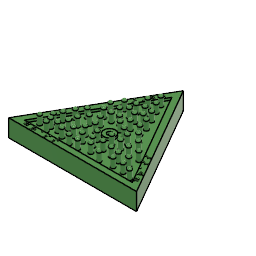
Piece Grass (Autodesk Fusion 360 design; units mm, degrees)
Autodesk Fusion 360 part; units mm, degrees
sketch "Sketch1" plane through (0, 0, 0) normal (0, 1, 0) x (1, 0, 0) in component "Peice Base"
  line L0 (0, 0) -> (69.85, 120.9837)
  line L1 (0, 0) -> (139.7, 0)
  line L2 (69.85, 120.9837) -> (139.7, 0)
  dimension "d1" = 139.7
  dimension "d2" = 139.7
  dimension "d4" = 139.7
  constraint coincident L0.start L1.start
  constraint horizontal L1
  measures "d1" distance of L0.start L0.end
  measures "d2" distance of L0.start L1.end
  measures "d4" distance of L0.end L1.end
extrude "Extrude1" add sketch "Sketch1" along normal blind 19.05 makes body 1 in component "Peice Base"
sketch "Sketch1 (2)" plane through (0, 0, 0) normal (0, 1, 0) x (1, 0, 0) in component "grass"
  line L0 (0, 0) -> (69.85, 120.9837)
  line L1 (0, 0) -> (139.7, 0)
  line L2 (69.85, 120.9837) -> (139.7, 0)
  dimension "d1_1" = 139.7
  dimension "d2_1" = 139.7
  dimension "d4_1" = 139.7
  constraint coincident L0.start L1.start
  constraint horizontal L1
  measures "d1_1" distance of L0.start L0.end
  measures "d2_1" distance of L0.start L1.end
  measures "d4_1" distance of L0.end L1.end
extrude "Extrude1'" add sketch "Sketch1 (2)" along normal blind 19.05 separate body makes body 2 in component "grass"
sketch "Sketch5" plane through (0, 19.05, 0) normal (0, 1, 0) x (-1, 0, 0) in component "grass"
  line L0 (0, 0) -> (-139.7, 0)
  line L1 (-139.7, 0) -> (-69.85, -120.9837)
  line L2 (-69.85, -120.9837) -> (0, 0)
  line L3 (-128.7015, -6.35) -> (-69.85, -108.2837)
  line L4 (-69.85, -108.2837) -> (-10.9985, -6.35)
  line L5 (-10.9985, -6.35) -> (-128.7015, -6.35)
  circle A0 centre (-69.85, -40.3279) radius 2.54
  circle A1 centre (-69.85, -40.3279) radius 6.35
  circle A2 centre (-69.537, -96.6095) radius 2.286
  circle A3 centre (-64.3272, -87.6271) radius 2.286
  circle A4 centre (-73.4892, -87.6271) radius 2.286
  circle A5 centre (-63.2493, -76.1296) radius 2.286
  circle A6 centre (-58.0395, -63.1949) radius 2.286
  circle A7 centre (-70.9742, -66.6083) radius 2.286
  circle A8 centre (-78.8787, -77.2075) radius 2.286
  circle A9 centre (-70.6149, -78.2854) radius 2.286
  circle A10 centre (-83.7292, -66.6083) radius 2.286
  circle A11 centre (-85.7053, -57.6258) radius 2.286
  circle A12 centre (-75.4654, -57.3169) radius 2.286
  circle A13 centre (-65.2254, -56.009) radius 2.286
  circle A14 centre (-49.596, -54.2125) radius 2.286
  circle A15 centre (-53.5483, -72.896) radius 2.286
  circle A16 centre (-40.4243, -45.4098) radius 2.286
  circle A17 centre (-55.7041, -44.5115) radius 2.286
  circle A18 centre (-79.4176, -46.6673) radius 2.286
  circle A19 centre (-92.1727, -49.7213) radius 2.286
  circle A20 centre (-58.9377, -35.7087) radius 2.286
  circle A21 centre (-48.1588, -40.0203) radius 2.286
  circle A22 centre (-34.925, -37.8645) radius 2.286
  circle A23 centre (-99.5383, -42.1761) radius 2.286
  circle A24 centre (-87.3222, -42.3557) radius 2.286
  circle A25 centre (-79.0583, -33.553) radius 2.286
  circle A26 centre (-88.7594, -33.553) radius 2.286
  circle A27 centre (-87.8611, -10.9173) radius 2.286
  circle A28 centre (-101.1551, -12.8934) radius 2.286
  circle A29 centre (-90.3762, -21.6962) radius 2.286
  circle A30 centre (-99.179, -31.7565) radius 2.286
  circle A31 centre (-99.3586, -20.4386) radius 2.286
  circle A32 centre (-112.1136, -12.8934) radius 2.286
  circle A33 centre (-109.4189, -21.8758) radius 2.286
  circle A34 centre (-109.4189, -32.8344) radius 2.286
  circle A35 centre (-121.4554, -10.558) radius 2.286
  circle A36 centre (-30.5533, -28.7025) radius 2.286
  circle A37 centre (-43.488, -31.9361) radius 2.286
  circle A38 centre (-56.4227, -27.2653) radius 2.286
  circle A39 centre (-67.7405, -29.0618) radius 2.286
  circle A40 centre (-80.1362, -22.9537) radius 2.286
  circle A41 centre (-75.4654, -14.3306) radius 2.286
  circle A42 centre (-70.7945, -21.1572) radius 2.286
  circle A43 centre (-61.0935, -19.3607) radius 2.286
  circle A44 centre (-64.6865, -10.558) radius 2.286
  circle A45 centre (-55.5244, -10.558) radius 2.286
  circle A46 centre (-51.0332, -19.8997) radius 2.286
  circle A47 centre (-41.5118, -23.852) radius 2.286
  circle A48 centre (-29.9275, -16.0295) radius 2.286
  circle A49 centre (-27.14, -21.6962) radius 2.286
  circle A50 centre (-37.7392, -15.9474) radius 2.286
  circle A51 centre (-45.2845, -12.8934) radius 2.286
  circle A52 centre (-71.1538, -50.6196) radius 2.286
  circle A53 centre (-47.9792, -63.1949) radius 2.286
  circle A54 centre (-76.7229, -70.2012) radius 2.286
  circle A55 centre (-57.6802, -54.3922) radius 2.286
  circle A56 centre (-63.2493, -68.5844) radius 2.286
  circle A57 centre (-20.5941, -13.3685) radius 2.286
  circle A58 centre (-30.8095, -10.3039) radius 2.286
  circle A59 centre (-14.8274, -5.4566) radius 0.7493
  circle A60 centre (-17.1134, -5.4566) radius 0.7493
  circle A61 centre (-17.1134, -3.1706) radius 0.7493
  circle A62 centre (-14.8274, -3.1706) radius 0.7493
  circle A63 centre (-23.2348, -5.4566) radius 0.7493
  circle A64 centre (-23.2348, -3.1706) radius 0.7493
  circle A65 centre (-23.2348, -0.8846) radius 0.7493
  circle A66 centre (-25.5208, -3.1706) radius 0.7493
  circle A67 centre (-31.6422, -5.4566) radius 0.7493
  circle A68 centre (-37.7636, -3.1706) radius 0.7493
  circle A69 centre (-37.7636, -0.8846) radius 0.7493
  circle A70 centre (-40.0496, -5.4566) radius 0.7493
  circle A71 centre (-40.0496, -5.4566) radius 0.7493
  circle A72 centre (-46.171, -3.1706) radius 0.7493
  circle A73 centre (-46.171, -0.8846) radius 0.7493
  circle A74 centre (-48.457, -5.4566) radius 0.7493
  circle A75 centre (-118.2703, -30.7774) radius 0.7493
  circle A76 centre (-115.1476, -31.6141) radius 0.7493
  circle A77 centre (-128.5954, -12.8938) radius 0.7493
  circle A78 centre (-116.0464, -39.2014) radius 0.7493
  circle A79 centre (-110.9439, -38.8951) radius 0.7493
  circle A80 centre (-125.5347, -18.195) radius 0.7493
  circle A81 centre (-119.3513, -24.3331) radius 0.7493
  circle A82 centre (-115.1476, -31.6141) radius 0.7493
  circle A83 centre (-129.7384, -10.914) radius 0.7493
  circle A84 centre (-120.2501, -31.9204) radius 0.7493
  circle A85 centre (-123.555, -17.052) radius 0.7493
  circle A86 centre (-126.6157, -11.7508) radius 0.7493
  circle A87 centre (-114.0666, -38.0584) radius 0.7493
  circle A88 centre (-124.3917, -20.1748) radius 0.7493
  circle A89 centre (-127.7587, -9.771) radius 0.7493
  circle A90 centre (-127.5145, -19.338) radius 0.7493
  circle A91 centre (-52.8628, -85.2716) radius 0.7493
  circle A92 centre (-53.6996, -82.1488) radius 0.7493
  circle A93 centre (-63.1879, -103.1551) radius 0.7493
  circle A94 centre (-46.6794, -79.1335) radius 0.7493
  circle A95 centre (-49.4959, -74.8678) radius 0.7493
  circle A96 centre (-60.1272, -97.8539) radius 0.7493
  circle A97 centre (-57.9033, -89.4298) radius 0.7493
  circle A98 centre (-53.6996, -82.1488) radius 0.7493
  circle A99 centre (-64.3309, -105.1349) radius 0.7493
  circle A100 centre (-50.8831, -86.4146) radius 0.7493
  circle A101 centre (-62.107, -96.7109) radius 0.7493
  circle A102 centre (-65.1677, -102.0121) radius 0.7493
  circle A103 centre (-48.6591, -77.9905) radius 0.7493
  circle A104 centre (-58.9842, -95.8741) radius 0.7493
  circle A105 centre (-66.3107, -103.9919) radius 0.7493
  circle A106 centre (-58.1475, -98.9969) radius 0.7493
  dimension "d22" = -6.35
  dimension "d40" = 5.08
  dimension "d41" = 69.85
  dimension "d42" = 40.3279
  dimension "d65" = 12.7
  dimension "d89" = 4.572
  dimension "d90" = 4.572
  dimension "d91" = 4.572
  dimension "d92" = 4.572
  dimension "d93" = 4.572
  dimension "d94" = 4.572
  dimension "d95" = 4.572
  dimension "d96" = 4.572
  dimension "d97" = 4.572
  dimension "d98" = 4.572
  dimension "d99" = 4.572
  dimension "d100" = 4.572
  dimension "d101" = 4.572
  dimension "d102" = 4.572
  dimension "d103" = 4.572
  dimension "d104" = 4.572
  dimension "d105" = 4.572
  dimension "d106" = 4.572
  dimension "d107" = 4.572
  dimension "d108" = 4.572
  dimension "d109" = 4.572
  dimension "d110" = 4.572
  dimension "d111" = 4.572
  dimension "d112" = 4.572
  dimension "d113" = 4.572
  dimension "d114" = 4.572
  dimension "d115" = 4.572
  dimension "d116" = 4.572
  dimension "d117" = 4.572
  dimension "d118" = 4.572
  dimension "d119" = 4.572
  dimension "d120" = 4.572
  dimension "d121" = 4.572
  dimension "d122" = 4.572
  dimension "d123" = 4.572
  dimension "d124" = 4.572
  dimension "d125" = 4.572
  dimension "d126" = 4.572
  dimension "d127" = 4.572
  dimension "d128" = 4.572
  dimension "d129" = 4.572
  dimension "d130" = 4.572
  dimension "d131" = 4.572
  dimension "d132" = 4.572
  dimension "d133" = 4.572
  dimension "d134" = 4.572
  dimension "d136" = 4.572
  dimension "d137" = 4.572
  dimension "d138" = 4.572
  dimension "d139" = 4.572
  dimension "d140" = 4.572
  dimension "d141" = 4.572
  dimension "d142" = 4.572
  dimension "d143" = 4.572
  dimension "d144" = 4.572
  dimension "d148" = 4.572
  dimension "d149" = 4.572
  dimension "d150" = 1.4986
  dimension "d151" = 1.4986
  dimension "d152" = 1.4986
  dimension "d153" = 1.4986
  dimension "d154" = 1.4986
  dimension "d155" = 1.4986
  dimension "d156" = 1.4986
  dimension "d157" = 1.4986
  dimension "d159" = 1.4986
  dimension "d160" = 1.4986
  dimension "d161" = 1.4986
  dimension "d163" = 1.4986
  dimension "d164" = 1.4986
  dimension "d166" = 1.4986
  dimension "d167" = 1.4986
  dimension "d169" = 1.4986
  dimension "d170" = 1.4986
  dimension "d171" = 1.4986
  dimension "d172" = 1.4986
  dimension "d173" = 1.4986
  dimension "d174" = 1.4986
  dimension "d175" = 1.4986
  dimension "d176" = 1.4986
  dimension "d177" = 1.4986
  dimension "d178" = 1.4986
  dimension "d179" = 1.4986
  dimension "d180" = 1.4986
  dimension "d181" = 1.4986
  dimension "d182" = 1.4986
  dimension "d183" = 1.4986
  dimension "d184" = 1.4986
  dimension "d185" = 1.4986
  dimension "d186" = 1.4986
  dimension "d187" = 1.4986
  dimension "d188" = 1.4986
  dimension "d189" = 1.4986
  dimension "d190" = 1.4986
  dimension "d191" = 1.4986
  dimension "d192" = 1.4986
  dimension "d193" = 1.4986
  dimension "d194" = 1.4986
  dimension "d195" = 1.4986
  dimension "d196" = 1.4986
  dimension "d197" = 1.4986
  dimension "d198" = 1.4986
  dimension "d199" = 1.4986
  dimension "d200" = 1.4986
  dimension "d201" = 1.4986
  constraint concentric A0 A1
  measures "d40" diameter of A0
  measures "d41" horizontal distance of L0.start A0.centre
  measures "d42" distance of L0 A0.centre
  measures "d65" diameter of A1
  measures "d89" diameter of A2
  measures "d90" diameter of A3
  measures "d91" diameter of A4
  measures "d92" diameter of A5
  measures "d93" diameter of A6
  measures "d94" diameter of A7
  measures "d95" diameter of A8
  measures "d96" diameter of A9
  measures "d97" diameter of A10
  measures "d98" diameter of A11
  measures "d99" diameter of A12
  measures "d100" diameter of A13
  measures "d101" diameter of A14
  measures "d102" diameter of A15
  measures "d103" diameter of A16
  measures "d104" diameter of A17
  measures "d105" diameter of A18
  measures "d106" diameter of A19
  measures "d107" diameter of A20
  measures "d108" diameter of A21
  measures "d109" diameter of A22
  measures "d110" diameter of A23
  measures "d111" diameter of A24
  measures "d112" diameter of A25
  measures "d113" diameter of A26
  measures "d114" diameter of A27
  measures "d115" diameter of A28
  measures "d116" diameter of A29
  measures "d117" diameter of A30
  measures "d118" diameter of A31
  measures "d119" diameter of A32
  measures "d120" diameter of A33
  measures "d121" diameter of A34
  measures "d122" diameter of A35
  measures "d123" diameter of A36
  measures "d124" diameter of A37
  measures "d125" diameter of A38
  measures "d126" diameter of A39
  measures "d127" diameter of A40
  measures "d128" diameter of A41
  measures "d129" diameter of A42
  measures "d130" diameter of A43
  measures "d131" diameter of A44
  measures "d132" diameter of A45
  measures "d133" diameter of A46
  measures "d134" diameter of A47
  measures "d136" diameter of A48
  measures "d137" diameter of A49
  measures "d138" diameter of A50
  measures "d139" diameter of A51
  measures "d140" diameter of A52
  measures "d141" diameter of A53
  measures "d142" diameter of A54
  measures "d143" diameter of A55
  measures "d144" diameter of A56
  measures "d148" diameter of A57
  measures "d149" diameter of A58
  measures "d150" diameter of A59
  measures "d151" diameter of A60
  measures "d152" diameter of A61
  measures "d153" diameter of A62
  measures "d154" diameter of A63
  measures "d155" diameter of A64
  measures "d156" diameter of A65
  measures "d157" diameter of A66
  measures "d159" diameter of A67
  measures "d160" diameter of A68
  measures "d161" diameter of A69
  measures "d163" diameter of A70
  measures "d164" diameter of A71
  measures "d166" diameter of A72
  measures "d167" diameter of A73
  measures "d169" diameter of A74
  measures "d170" diameter of A89
  measures "d171" diameter of A86
  measures "d172" diameter of A77
  measures "d173" diameter of A83
  measures "d174" diameter of A85
  measures "d175" diameter of A80
  measures "d176" diameter of A90
  measures "d177" diameter of A88
  measures "d178" diameter of A81
  measures "d179" diameter of A75
  measures "d180" diameter of A84
  measures "d181" diameter of A76
  measures "d182" diameter of A82
  measures "d183" diameter of A87
  measures "d184" diameter of A78
  measures "d185" diameter of A79
  measures "d186" diameter of A105
  measures "d187" diameter of A102
  measures "d188" diameter of A93
  measures "d189" diameter of A99
  measures "d190" diameter of A101
  measures "d191" diameter of A96
  measures "d192" diameter of A106
  measures "d193" diameter of A104
  measures "d194" diameter of A97
  measures "d195" diameter of A91
  measures "d196" diameter of A100
  measures "d197" diameter of A92
  measures "d198" diameter of A98
  measures "d199" diameter of A103
  measures "d200" diameter of A94
  measures "d201" diameter of A95
extrude "Extrude7" cut sketch "Sketch5" against normal blind 3.048 contours A0 bodies 2 in component "grass"
extrude "Extrude8" cut sketch "Sketch5" against normal blind 2.54 contours L3 L4 L5 bodies 2 in component "grass"
extrude "Extrude9" add sketch "Sketch5" along normal blind 8.89 contours A2 | A3 | A4 | A5 | A6 | A7 | A8 | A9 | A10 | A11 | A12 | A13 | A14 | A15 | A16 | A17 | A18 | A19 | A20 | A21 | A22 | A23 | A24 | A25 | A26 | A27 | A28 | A29 | A30 | A31 | A32 | A33 | A34 | A35 | A36 | A37 | A38 | A39 | A40 | A41 | A42 | A43 | A44 | A45 | A46 | A47 | A48 | A49 | A50 | A51 | A52 | A53 | A54 | A55 | A56 | A57 | A58 bodies 2 in component "grass"
fillet "Fillet1" radius 2.286 57 edges at (123.5867, 27.94, -11.3846) (114.2449, 27.94, -13.7201) (103.2864, 27.94, -13.7201) (89.9924, 27.94, -11.7439) (77.5967, 27.94, -15.1572) (66.8178, 27.94, -11.3846) (57.6557, 27.94, -11.3846) (63.2248, 27.94, -20.1874) (72.9258, 27.94, -21.9839) (82.2675, 27.94, -23.7804) (92.5075, 27.94, -22.5228) (101.4899, 27.94, -21.2653) (111.5502, 27.94, -22.7025) (111.5502, 27.94, -33.661) (101.3103, 27.94, -32.5831) (90.8907, 27.94, -34.3796) (89.4535, 27.94, -43.1824) (94.304, 27.94, -50.548) (101.6696, 27.94, -43.0027) (87.8366, 27.94, -58.4525) (85.8605, 27.94, -67.4349) (77.5967, 27.94, -58.1435) (81.1896, 27.94, -34.3796) (69.8718, 27.94, -29.8884) (58.554, 27.94, -28.0919) (53.1645, 27.94, -20.7263) (47.4158, 27.94, -13.7201) (32.9408, 27.94, -11.1306) (32.0588, 27.94, -16.8562) (22.7254, 27.94, -14.1952) (29.2713, 27.94, -22.5228) (32.6846, 27.94, -29.5291) (43.6431, 27.94, -24.6786) (39.8705, 27.94, -16.7741) (45.6193, 27.94, -32.7628) (37.0563, 27.94, -38.6912) (42.5556, 27.94, -46.2364) (50.2901, 27.94, -40.847) (57.8354, 27.94, -45.3382) (61.069, 27.94, -36.5354) (51.7273, 27.94, -55.0392) (50.1105, 27.94, -64.0216) (60.1708, 27.94, -64.0216) (59.8115, 27.94, -55.2188) (55.6796, 27.94, -73.7226) (67.3567, 27.94, -56.8357) (73.2851, 27.94, -51.4462) (81.5489, 27.94, -47.4939) (73.1055, 27.94, -67.4349) (65.3806, 27.94, -69.411) (65.3806, 27.94, -76.9563) (66.4585, 27.94, -88.4538) (75.6205, 27.94, -88.4538) (72.7462, 27.94, -79.1121) (81.01, 27.94, -78.0342) (78.8542, 27.94, -71.0279) (71.6683, 27.94, -97.4362) on bodies 2 in component "grass"
extrude "Extrude10" add sketch "Sketch5" along normal blind 0.762 contours A59 | A60 | A61 | A62 | A63 | A64 | A65 | A66 | A67 | A68 | A69 | A70 A71 | A72 | A73 | A74 | A75 | A76 A82 | A77 | A78 | A79 | A80 | A81 | A83 | A84 | A85 | A86 | A87 | A88 | A89 | A90 | A91 | A92 A98 | A93 | A94 | A95 | A96 | A97 | A99 | A100 | A101 | A102 | A103 | A104 | A105 | A106 bodies 2 in component "grass"
fillet "Fillet2" radius 0.7493 45 edges at (66.196, 19.812, -103.2514) (65.053, 19.812, -101.2717) (63.0733, 19.812, -102.4147) (64.2163, 19.812, -104.3944) (61.9923, 19.812, -95.9704) (58.8696, 19.812, -95.1336) (60.0126, 19.812, -97.1134) (58.0329, 19.812, -98.2564) (57.7886, 19.812, -88.6894) (50.7685, 19.812, -85.6741) (52.7482, 19.812, -84.5311) (53.5849, 19.812, -81.4083) (46.5648, 19.812, -78.393) (48.5445, 19.812, -77.25) (49.3812, 19.812, -74.1273) (127.1748, 19.812, -10.2405) (129.1545, 19.812, -11.3835) (128.0115, 19.812, -13.3633) (126.0318, 19.812, -12.2203) (122.9711, 19.812, -17.5216) (124.9508, 19.812, -18.6646) (126.9305, 19.812, -19.8076) (123.8078, 19.812, -20.6443) (118.7674, 19.812, -24.8026) (114.5637, 19.812, -32.0836) (117.6864, 19.812, -31.2469) (119.6661, 19.812, -32.3899) (115.4624, 19.812, -39.6709) (113.4827, 19.812, -38.5279) (110.36, 19.812, -39.3646) (15.526, 19.812, -3.4416) (17.812, 19.812, -3.4416) (17.812, 19.812, -5.7276) (15.526, 19.812, -5.7276) (23.9334, 19.812, -5.7276) (23.9334, 19.812, -3.4416) (26.2194, 19.812, -3.4416) (23.9334, 19.812, -1.1556) (32.3408, 19.812, -5.7276) (38.4622, 19.812, -3.4416) (40.7482, 19.812, -5.7276) (38.4622, 19.812, -1.1556) (46.8696, 19.812, -3.4416) (49.1556, 19.812, -5.7276) (46.8696, 19.812, -1.1556) on bodies 2 in component "grass"
component "Peice Base" placed x (1, 0, 0) y (0, 1, 0) z (0, 0, 1) at (0, 0, 0)
component "grass" placed x (1, 0, 0) y (0, 1, 0) z (0, 0, 1) at (0, 0, 0)
